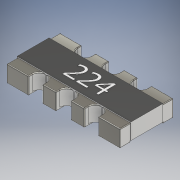
# Autodesk Inventor part: ResistorArray-1632
Saved by Autodesk Inventor 2018 (Build 220112000, 112)
## iProperties
Created: 2018-09-29
Part Number: ResistorArray-1632
Material: Copper
Document SubType Name: Modeling
Designer: Bradley
Density: 8.94 g/cm^3
Appearance: Smooth - White
Author: Bradley
Autodesk Inventor part; units mm, degrees
ref_plane "YZ Plane" through (0, 0, 0) normal (1, 0, 0) x (0, 1, 0)
ref_plane "XZ Plane" through (0, 0, 0) normal (0, 1, 0) x (-1, 0, 0)
ref_plane "XY Plane" through (0, 0, 0) normal (0, 0, 1) x (1, 0, 0)
sketch "Sketch1" plane through (0, 0, 0) normal (0, 0, 1) x (1, 0, 0)
  line L0 (-1.6, -0.45) -> (1.6, -0.45)
  line L1 (1.6, -0.45) -> (1.6, 0.45)
  line L2 (1.6, 0.45) -> (-1.6, 0.45)
  line L3 (-1.6, 0.45) -> (-1.6, -0.45)
  line L4 (-1.6, -0.45) -> (1.6, 0.45) construction
  line L5 (1.6, -0.45) -> (-1.6, 0.45) construction
  point P0 (0, 0)
  dimension "d0" = 3.2
  dimension "d1" = 0.9
  constraints: 12 end point, 2 midpoint, 2 parallel, 1 horizontal, 1 perpendicular
  measures "d0" distance of L2.end L1.end
  measures "d1" distance of L2.end L0.start
extrude "Extrusion1" add sketch "Sketch1" along normal mid plane 0.45
sketch "Sketch2" plane through (0, 0, 0) normal (0, 0, 1) x (1, 0, 0)
  line L0 (-1.6, -0.45) -> (1.6, -0.45) projected
  line L1 (1.6, -0.45) -> (1.6, 0.45) projected
  line L2 (1.6, 0.45) -> (-1.6, 0.45) projected
  line L3 (-1.6, 0.45) -> (-1.6, -0.45) projected
  line L4 (1.6, 0.45) -> (-1.6, 0.45) projected
  line L5 (-1.59, 0.45) -> (-0.98, 0.45)
  line L6 (-0.98, 0.45) -> (-0.98, 0.75)
  line L7 (-0.98, 0.75) -> (-1.59, 0.75)
  line L8 (-1.59, 0.75) -> (-1.59, 0.45)
  line L9 (1.59, -0.45) -> (0.98, -0.45)
  line L10 (0.98, -0.45) -> (0.98, -0.75)
  line L11 (0.98, -0.75) -> (1.59, -0.75)
  line L12 (1.59, -0.75) -> (1.59, -0.45)
  line L13 (1.59, 0.45) -> (0.98, 0.45)
  line L14 (0.98, 0.45) -> (0.98, 0.75)
  line L15 (0.98, 0.75) -> (1.59, 0.75)
  line L16 (1.59, 0.75) -> (1.59, 0.45)
  line L17 (-0.59, 0.45) -> (-0.21, 0.45)
  line L18 (-0.21, 0.45) -> (-0.21, 0.75)
  line L19 (-0.21, 0.75) -> (-0.59, 0.75)
  line L20 (-0.59, 0.75) -> (-0.59, 0.45)
  line L21 (-1.6, -0.45) -> (1.6, -0.45) projected
  line L22 (-0.59, -0.45) -> (-0.21, -0.45)
  line L23 (-0.21, -0.45) -> (-0.21, -0.75)
  line L24 (-0.21, -0.75) -> (-0.59, -0.75)
  line L25 (-0.59, -0.75) -> (-0.59, -0.45)
  line L26 (0.21, -0.45) -> (0.59, -0.45)
  line L27 (0.59, -0.45) -> (0.59, -0.75)
  line L28 (0.59, -0.75) -> (0.21, -0.75)
  line L29 (0.21, -0.75) -> (0.21, -0.45)
  line L30 (0.59, 0.75) -> (0.21, 0.75)
  line L31 (0.21, 0.75) -> (0.21, 0.45)
  line L32 (0.59, 0.45) -> (0.59, 0.75)
  line L33 (0.21, 0.45) -> (0.59, 0.45)
  line L34 (1.6, -0.45) -> (-1.6, -0.45) projected
  line L35 (-1.59, -0.45) -> (-0.98, -0.45)
  line L36 (-0.98, -0.45) -> (-0.98, -0.75)
  line L37 (-0.98, -0.75) -> (-1.59, -0.75)
  line L38 (-1.59, -0.75) -> (-1.59, -0.45)
  point P0 (0, 0)
  point P1 (0.4, 0.75)
  dimension "d4" = 0.61
  dimension "d5" = 0.38
  dimension "d9" = 0.8
  dimension "d18" = 0.01
  dimension "d19" = 0.01
  dimension "d25" = 0.4
  dimension "d26" = 1.5
  constraints: 64 end point, 12 parallel, 10 collinear, 10 point on line, 7 horizontal, 6 perpendicular, 1 midpoint, 17 other
  measures "d4" distance of L6.end L7.end
  measures "d5" distance of L18.end L19.end
  measures "d9" distance of L22.end L26.end
  measures "d18" distance between parallel lines of L1 L16
  measures "d19" distance between parallel lines of L3 L8
  measures "d25" horizontal distance of point (0, 0) point (0.4, 0.75)
  measures "d26" distance between parallel lines of L37 L7
extrude "Extrusion2" add sketch "Sketch2" along normal blind 0.2 and the other way blind 0.275 contours L0 L36 L37 L38 | L8 L7 L6 L2 | L0 L23 L24 L25 | L20 L19 L18 L2 | L0 L27 L28 L29 | L31 L30 L32 L2 | L0 L12 L11 L10 | L14 L15 L16 L2
fillet "Fillet2" radius 0.19 12 edges at (-0.98, -0.45, -0.0125) (-0.59, -0.45, -0.0125) (-0.21, -0.45, -0.0125) (0.21, -0.45, -0.0125) (0.59, -0.45, -0.0125) (0.98, -0.45, -0.0125) (-0.98, 0.45, -0.0125) (-0.59, 0.45, -0.0125) (-0.21, 0.45, -0.0125) (0.21, 0.45, -0.0125) (0.59, 0.45, -0.0125) (0.98, 0.45, -0.0125)
fillet "Fillet1" radius 0.02 88 edges at (0.98, 0.45, -0.25) (1.285, 0.45, -0.275) (1.59, 0.45, -0.25) (1.59, 0.6, -0.275) (0.98, 0.6, -0.275) (1.285, 0.75, -0.275) (0.98, 0.695, 0.2) (0.98, 0.75, -0.0375) (1.285, 0.75, 0.2) (1.59, 0.75, -0.0375) (1.59, 0.6, 0.2) (1.285, -0.45, -0.275) (1.59, -0.6, -0.275) (1.285, -0.75, -0.275) (0.98, -0.6, -0.275) (1.59, -0.6, 0.2) (1.59, -0.75, -0.0375) (1.59, -0.45, -0.25) (1.285, -0.75, 0.2) (0.98, -0.75, -0.0375) (0.98, -0.695, 0.2) (0.98, -0.45, -0.25) (0.4, -0.45, -0.275) (0.59, -0.6, -0.275) (0.4, -0.75, -0.275) (0.21, -0.6, -0.275) (0.59, -0.695, 0.2) (0.59, -0.75, -0.0375) (0.59, -0.45, -0.25) (0.4, -0.75, 0.2) (0.21, -0.75, -0.0375) (0.21, -0.695, 0.2) (0.21, -0.45, -0.25) (-0.21, -0.45, -0.25) (-0.4, -0.45, -0.275) (-0.59, -0.45, -0.25) (-0.59, -0.6, -0.275) (-0.21, -0.6, -0.275) (-0.4, -0.75, -0.275) (-0.21, -0.695, 0.2) (-0.21, -0.75, -0.0375) (-0.4, -0.75, 0.2) (-0.59, -0.75, -0.0375) (-0.59, -0.695, 0.2) (-0.4, 0.45, -0.275) (-0.59, 0.6, -0.275) (-0.4, 0.75, -0.275) (-0.21, 0.6, -0.275) (-0.59, 0.695, 0.2) (-0.59, 0.75, -0.0375) (-0.59, 0.45, -0.25) (-0.4, 0.75, 0.2) (-0.21, 0.75, -0.0375) (-0.21, 0.695, 0.2) (-0.21, 0.45, -0.25) (0.4, 0.45, -0.275) (0.21, 0.6, -0.275) (0.4, 0.75, -0.275) (0.59, 0.6, -0.275) (0.21, 0.695, 0.2) (0.21, 0.75, -0.0375) (0.21, 0.45, -0.25) (0.4, 0.75, 0.2) (0.59, 0.75, -0.0375) (0.59, 0.695, 0.2) (0.59, 0.45, -0.25) (-1.285, 0.45, -0.275) (-1.59, 0.6, -0.275) (-1.285, 0.75, -0.275) (-0.98, 0.6, -0.275) (-1.59, 0.6, 0.2) (-1.59, 0.75, -0.0375) (-1.59, 0.45, -0.25) (-1.285, 0.75, 0.2) (-0.98, 0.75, -0.0375) (-0.98, 0.695, 0.2) (-0.98, 0.45, -0.25) (-0.98, -0.45, -0.25) (-1.285, -0.45, -0.275) (-1.59, -0.45, -0.25) (-1.59, -0.6, -0.275) (-0.98, -0.6, -0.275) (-1.285, -0.75, -0.275) (-0.98, -0.695, 0.2) (-0.98, -0.75, -0.0375) (-1.285, -0.75, 0.2) (-1.59, -0.75, -0.0375) (-1.59, -0.6, 0.2)
sketch "Sketch4" plane through (0, 0, 0.225) normal (0, 0, 1) x (1, 0, 0)
  line L0 (-1.6, -0.45) -> (1.6, -0.45) construction
  line L1 (1.6, -0.45) -> (1.6, 0.45) construction
  line L2 (1.6, 0.45) -> (-1.6, 0.45) construction
  line L3 (-1.6, 0.45) -> (-1.6, -0.45) construction
  line L4 (-1.6, -0.45) -> (-1.6, 0.45) construction
  line L5 (-1.6, 0) -> (1.6, 0) construction
  line L6 (-0.218, -0.25) -> (-0.5263, -0.25)
  line L7 (-0.5263, -0.25) -> (-0.5263, -0.1791)
  spline S0 degree 2 poles (-0.5263, -0.1791) (-0.4931, -0.1479) (-0.434, -0.09) (-0.4056, -0.0588) knots 0 0 0 1 2 2 2
  spline S1 degree 2 poles (-0.4056, -0.0588) (-0.3485, 0.0041) (-0.3067, 0.0794) (-0.3067, 0.1195) knots 0 0 0 1 2 2 2
  spline S2 degree 2 poles (-0.3067, 0.1195) (-0.3067, 0.1406) (-0.3197, 0.1722) (-0.3314, 0.1823) knots 0 0 0 1 2 2 2
  spline S3 degree 2 poles (-0.3314, 0.1823) (-0.3432, 0.1925) (-0.374, 0.2026) (-0.3926, 0.2026) knots 0 0 0 1 2 2 2
  spline S4 degree 2 poles (-0.3926, 0.2026) (-0.4105, 0.2026) (-0.4469, 0.1937) (-0.4635, 0.1868) knots 0 0 0 1 2 2 2
  spline S5 degree 2 poles (-0.4635, 0.1868) (-0.4777, 0.1811) (-0.5041, 0.1649) (-0.5122, 0.1592) knots 0 0 0 1 2 2 2
  line L8 (-0.5122, 0.1592) -> (-0.5158, 0.1592)
  line L9 (-0.5158, 0.1592) -> (-0.5158, 0.2306)
  spline S6 degree 2 poles (-0.5158, 0.2306) (-0.4951, 0.2407) (-0.421, 0.2605) (-0.3878, 0.2605) knots 0 0 0 1 2 2 2
  spline S7 degree 2 poles (-0.3878, 0.2605) (-0.3177, 0.2605) (-0.2387, 0.1864) (-0.2387, 0.1232) knots 0 0 0 1 2 2 2
  spline S8 degree 2 poles (-0.2387, 0.1232) (-0.2387, 0.0936) (-0.2524, 0.0442) (-0.2646, 0.0231) knots 0 0 0 1 2 2 2
  spline S9 degree 2 poles (-0.2646, 0.0231) (-0.2767, 0.0012) (-0.312, -0.0417) (-0.3314, -0.0624) knots 0 0 0 1 2 2 2
  spline S10 degree 2 poles (-0.3314, -0.0624) (-0.363, -0.0968) (-0.4404, -0.1706) (-0.4635, -0.1921) knots 0 0 0 1 2 2 2
  line L10 (-0.4635, -0.1921) -> (-0.218, -0.1921)
  line L11 (-0.218, -0.1921) -> (-0.218, -0.25)
  line L12 (0.1572, -0.25) -> (-0.1511, -0.25)
  line L13 (-0.1511, -0.25) -> (-0.1511, -0.1791)
  spline S11 degree 2 poles (-0.1511, -0.1791) (-0.1179, -0.1479) (-0.0588, -0.09) (-0.0304, -0.0588) knots 0 0 0 1 2 2 2
  spline S12 degree 2 poles (-0.0304, -0.0588) (0.0267, 0.0041) (0.0685, 0.0794) (0.0685, 0.1195) knots 0 0 0 1 2 2 2
  spline S13 degree 2 poles (0.0685, 0.1195) (0.0685, 0.1406) (0.0555, 0.1722) (0.0438, 0.1823) knots 0 0 0 1 2 2 2
  spline S14 degree 2 poles (0.0438, 0.1823) (0.032, 0.1925) (0.0012, 0.2026) (-0.0174, 0.2026) knots 0 0 0 1 2 2 2
  spline S15 degree 2 poles (-0.0174, 0.2026) (-0.0353, 0.2026) (-0.0717, 0.1937) (-0.0883, 0.1868) knots 0 0 0 1 2 2 2
  spline S16 degree 2 poles (-0.0883, 0.1868) (-0.1025, 0.1811) (-0.1288, 0.1649) (-0.137, 0.1592) knots 0 0 0 1 2 2 2
  line L14 (-0.137, 0.1592) -> (-0.1406, 0.1592)
  line L15 (-0.1406, 0.1592) -> (-0.1406, 0.2306)
  spline S17 degree 2 poles (-0.1406, 0.2306) (-0.1199, 0.2407) (-0.0458, 0.2605) (-0.0126, 0.2605) knots 0 0 0 1 2 2 2
  spline S18 degree 2 poles (-0.0126, 0.2605) (0.0575, 0.2605) (0.1365, 0.1864) (0.1365, 0.1232) knots 0 0 0 1 2 2 2
  spline S19 degree 2 poles (0.1365, 0.1232) (0.1365, 0.0936) (0.1228, 0.0442) (0.1106, 0.0231) knots 0 0 0 1 2 2 2
  spline S20 degree 2 poles (0.1106, 0.0231) (0.0985, 0.0012) (0.0632, -0.0417) (0.0438, -0.0624) knots 0 0 0 1 2 2 2
  spline S21 degree 2 poles (0.0438, -0.0624) (0.0122, -0.0968) (-0.0652, -0.1706) (-0.0883, -0.1921) knots 0 0 0 1 2 2 2
  line L16 (-0.0883, -0.1921) -> (0.1572, -0.1921)
  line L17 (0.1572, -0.1921) -> (0.1572, -0.25)
  line L18 (0.5458, -0.0782) -> (0.4862, -0.0782)
  line L19 (0.4862, -0.0782) -> (0.4862, -0.25)
  line L20 (0.4862, -0.25) -> (0.4218, -0.25)
  line L21 (0.4218, -0.25) -> (0.4218, -0.0782)
  line L22 (0.4218, -0.0782) -> (0.201, -0.0782)
  line L23 (0.201, -0.0782) -> (0.201, -0.0077)
  line L24 (0.201, -0.0077) -> (0.4246, 0.25)
  line L25 (0.4246, 0.25) -> (0.4862, 0.25)
  line L26 (0.4862, 0.25) -> (0.4862, -0.0243)
  line L27 (0.4862, -0.0243) -> (0.5458, -0.0243)
  line L28 (0.5458, -0.0243) -> (0.5458, -0.0782)
  line L29 (0.4218, -0.0243) -> (0.4218, 0.171)
  line L30 (0.4218, 0.171) -> (0.2536, -0.0243)
  line L31 (0.2536, -0.0243) -> (0.4218, -0.0243)
  point P0 (0, 0)
  constraints: 2 end point, 2 midpoint, 1 horizontal
extrude "Extrusion4" add sketch "Sketch4" along normal blind 0.01
equation "\"d19\" = d18"
equation "\"d25\" = 0.5 * d9"
body "Solid1"
